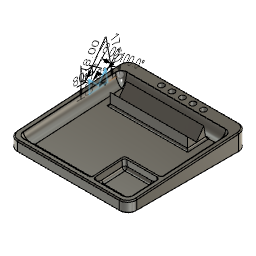
Rolling Tray with Mixer (Autodesk Fusion 360 design; units mm, degrees)
Autodesk Fusion 360 part; units mm, degrees
sketch "Esquisse2" plane through (0, 0, 0) normal (1, 0, 0) x (0, 1, 0)
  line L0 (0, 0) -> (170, 0)
  line L1 (170, 0) -> (170, 25)
  line L2 (0, 0) -> (0, 15)
  line L3 (170, 25) -> (0, 15)
  dimension "d3" = 170
  dimension "d4" = 15
  constraint coincident L0.start L2.start
  constraint horizontal L0
  constraint perpendicular L0 L1
  constraint vertical L2
  measures "d3" distance of L0.start L0.end
  measures "d4" distance of L0.start L2.end
extrude "Extrusion1" add sketch "Esquisse2" along normal blind 170
fillet "Congé1" radius 12.5 4 edges at (0, 170, 12.5) (0, 0, 7.5) (170, 0, 7.5) (170, 170, 12.5)
chamfer "Chanfrein1" distance 1.5 angle 45 16 edges at (85, 170, 25) (166.3388, 166.3388, 24.7846) (170, 85, 20) (166.3388, 3.6612, 15.2154) (85, 0, 15) (3.6612, 3.6612, 15.2154) (0, 85, 20) (3.6612, 166.3388, 24.7846) (0, 85, 0) (3.6612, 166.3388, 0) (85, 170, 0) (166.3388, 166.3388, 0) (170, 85, 0) (166.3388, 3.6612, 0) (85, 0, 0) (3.6612, 3.6612, 0)
sketch "Esquisse3" plane through (0, -0.8793, 14.9483) normal (0, -0.058722, 0.998274) x (1, 0, 0)
  line L0 (1.5, 158.5649) -> (1.5, 13.4024)
  spline S0 degree 3 poles (1.5003, 13.3248) (1.5002, 13.3377) (1.5001, 13.3506) (1.5, 13.3765) (1.5, 13.3895) (1.5, 13.4024) knots 1.56375 1.56375 1.56375 1.56375 1.567273 1.567273 1.570796 1.570796 1.570796 1.570796
  spline S1 degree 3 poles (12.5, 2.3808) (10.7152, 2.3808) (8.932, 2.8244) (6.3871, 4.174) (5.4968, 4.8327) (4.7227, 5.6081) (3.9487, 6.3835) (3.291, 7.2754) (1.9553, 9.8029) (1.5127, 11.5616) (1.5003, 13.3248) knots 0 0 0 0 0.486881 0.486881 0.785398 0.785398 0.785398 1.083915 1.083915 1.56375 1.56375 1.56375 1.56375
  line L1 (12.5, 2.3808) -> (157.5, 2.3808)
  spline S2 degree 3 poles (168.4997, 13.3248) (168.4873, 11.5616) (168.0447, 9.8029) (166.709, 7.2754) (166.0513, 6.3835) (165.2773, 5.6081) (164.5032, 4.8327) (163.6129, 4.174) (161.068, 2.8244) (159.2848, 2.3808) (157.5, 2.3808) knots -1.56375 -1.56375 -1.56375 -1.56375 -1.083915 -1.083915 -0.785398 -0.785398 -0.785398 -0.486881 -0.486881 0 0 0 0
  spline S3 degree 3 poles (168.5, 13.4024) (168.5, 13.3895) (168.5, 13.3765) (168.4999, 13.3506) (168.4998, 13.3377) (168.4997, 13.3248) knots -1.570796 -1.570796 -1.570796 -1.570796 -1.567273 -1.567273 -1.56375 -1.56375 -1.56375 -1.56375
  line L2 (168.5, 13.4024) -> (168.5, 158.5649)
  line L3 (168.5, 158.6531) -> (168.5, 158.5649)
  spline S4 degree 3 poles (157.5, 169.6747) (159.2794, 169.6747) (161.0571, 169.2338) (163.6041, 167.888) (164.4993, 167.2267) (165.2773, 166.4475) (166.0552, 165.6682) (166.7155, 164.7712) (168.0595, 162.2188) (168.5, 160.4367) (168.5, 158.6531) knots 0 0 0 0 0.485398 0.485398 0.785398 0.785398 0.785398 1.085399 1.085399 1.570796 1.570796 1.570796 1.570796
  line L4 (157.5, 169.6747) -> (12.5, 169.6747)
  spline S5 degree 3 poles (1.5, 158.6531) (1.5, 160.4367) (1.9405, 162.2188) (3.2845, 164.7712) (3.9448, 165.6682) (4.7227, 166.4475) (5.5007, 167.2267) (6.3959, 167.888) (8.9429, 169.2338) (10.7206, 169.6747) (12.5, 169.6747) knots -1.570796 -1.570796 -1.570796 -1.570796 -1.085399 -1.085399 -0.785398 -0.785398 -0.785398 -0.485398 -0.485398 0 0 0 0
  line L5 (1.5, 158.5649) -> (1.5, 158.6531)
  line L6 (163.5, 7.3808) -> (6.5, 7.3808)
  line L7 (6.5, 7.3808) -> (6.5, 154.6747)
  line L8 (6.5, 154.6747) -> (163.5, 154.6747)
  line L9 (163.5, 154.6747) -> (163.5, 7.3808)
  line L10 (163.5, 7.3808) -> (6.5, 154.6747) construction
  line L11 (6.5, 7.3808) -> (163.5, 154.6747) construction
  point P0 (85, 81.0278)
  dimension "d10" = 5
  dimension "d11" = 5
  dimension "d12" = 5
  dimension "d13" = 15
  constraint horizontal L6
  constraint perpendicular L6 L7
  constraint parallel L6 L8
  constraint parallel L7 L9
  constraint coincident L10 P0
  constraint coincident L11 P0
  measures "d10" distance of L1 L6
  measures "d11" distance of L2 L9
  measures "d12" distance of L0 L7
  measures "d13" distance of L4 L8
extrude "Extrusion2" cut sketch "Esquisse3" against normal blind 12.5 contours L6 L7 L8 L9
fillet "Congé2" radius 8 4 edges at (163.5, 153.8955, 17.7919) (163.5, 6.8558, 9.1425) (6.5, 6.8558, 9.1425) (6.5, 153.8955, 17.7919)
fillet "Congé4" radius 12 8 edges at (8.8431, 9.5619, 3.0409) (6.5, 80.7427, 7.228) (8.8431, 151.9234, 11.4151) (85, 154.2625, 11.5527) (161.1569, 151.9234, 11.4151) (163.5, 80.7427, 7.228) (161.1569, 9.5619, 3.0409) (85, 7.2228, 2.9033)
sketch "Esquisse5" plane through (0, 0, 0) normal (0, 0, -1) x (1, 0, 0)
  line L0 (1.5, -12.5) -> (1.5, -157.5)
  arc A0 (1.5, -157.5) -> (12.5, -168.5) centre (12.5, -157.5) ccw
  line L1 (12.5, -168.5) -> (157.5, -168.5)
  arc A1 (157.5, -168.5) -> (168.5, -157.5) centre (157.5, -157.5) ccw
  line L2 (168.5, -157.5) -> (168.5, -12.5)
  arc A2 (168.5, -12.5) -> (157.5, -1.5) centre (157.5, -12.5) ccw
  line L3 (157.5, -1.5) -> (12.5, -1.5)
  arc A3 (12.5, -1.5) -> (1.5, -12.5) centre (12.5, -12.5) ccw
  circle A4 centre (86.5, -161) radius 4
  circle A5 centre (101.5, -161) radius 4
  circle A6 centre (71.5, -161) radius 4
  circle A7 centre (116.5, -161) radius 4
  circle A8 centre (56.5, -161) radius 4
  dimension "d60" = 8
  dimension "d67" = 8
  dimension "d68" = 8
  dimension "d69" = 8
  dimension "d70" = 8
  measures "d60" diameter of A4
  measures "d67" diameter of A5
  measures "d68" diameter of A6
  measures "d69" diameter of A7
  measures "d70" diameter of A8
extrude "Extrusion3" cut sketch "Esquisse5" against normal blind 15 from surface at -10 contours A4 | A5 | A6 | A7 | A8
sketch "Esquisse6" plane through (0, 0, 0) normal (1, 0, 0) x (0, 1, 0)
  line L0 (140.9646, 10.5002) -> (137.9258, 27.7343)
  line L1 (140.9646, 10.5002) -> (159.1172, 10.5002) construction
  line L2 (137.9258, 27.7343) -> (127.6014, 12.9896)
  line L3 (127.6014, 12.9896) -> (114.8735, 25.7175)
  line L4 (114.8735, 25.7175) -> (114.8735, 8.2175)
  line L5 (140.9646, 10.5002) -> (114.8735, 8.2175)
  dimension "d47" = 100
  dimension "d48" = 80
  dimension "d49" = 45
  dimension "d50" = 17.5
  dimension "d51" = 17.5
  dimension "d52" = 18
  dimension "d53" = 18
  constraint horizontal L1
  constraint vertical L4
  measures "d47" angle of L0 L1
  measures "d48" angle of L2 L3
  measures "d49" angle of L0 L2
  measures "d50" distance of L0.start L0.end
  measures "d51" distance of L3.end L4.end
  measures "d52" distance of L0.end L2.end
  measures "d53" distance of L2.end L3.end
extrude "Extrusion4" add sketch "Esquisse6" along normal blind 110 from surface at 30
fillet "Congé5" radius 2.5 4 edges at (85, 114.8735, 9.2357) (140, 127.8955, 10.0017) (85, 140.9175, 10.7677) (30, 127.8955, 10.0017)
sketch "Esquisse8" plane through (0, -0.8793, 14.9483) normal (0, -0.058722, 0.998274) x (1, 0, 0)
  ellipse E0 centre (56.5, 162.1591) end of major axis (56.5, 166.1661) minor radius 4
  ellipse E1 centre (71.5, 162.1591) end of major axis (71.5, 166.1661) minor radius 4
  ellipse E2 centre (101.5, 162.1591) end of major axis (101.5, 166.1661) minor radius 4
  ellipse E3 centre (86.5, 162.1591) end of major axis (86.5, 166.1661) minor radius 4
  ellipse E4 centre (116.5, 162.1591) end of major axis (116.5, 166.1661) minor radius 4
  line L0 (6.5, 15.3808) -> (6.5, 146.6747)
  arc A0 (14.5, 154.6747) -> (6.5, 146.6747) centre (14.5, 146.6747) ccw
  line L1 (14.5, 154.6747) -> (155.5, 154.6747)
  arc A1 (163.5, 146.6747) -> (155.5, 154.6747) centre (155.5, 146.6747) ccw
  line L2 (163.5, 146.6747) -> (163.5, 15.3808)
  arc A2 (155.5, 7.3808) -> (163.5, 15.3808) centre (155.5, 15.3808) ccw
  line L3 (155.5, 7.3808) -> (14.5, 7.3808)
  arc A3 (6.5, 15.3808) -> (14.5, 7.3808) centre (14.5, 15.3808) ccw
  line L4 (1.5, 158.5649) -> (1.5, 13.4024)
  spline S0 degree 3 poles (1.5003, 13.3248) (1.5002, 13.3377) (1.5001, 13.3506) (1.5, 13.3765) (1.5, 13.3895) (1.5, 13.4024) knots 1.56375 1.56375 1.56375 1.56375 1.567273 1.567273 1.570796 1.570796 1.570796 1.570796
  spline S1 degree 3 poles (12.5, 2.3808) (10.7152, 2.3808) (8.932, 2.8244) (6.3871, 4.174) (5.4968, 4.8327) (4.7227, 5.6081) (3.9487, 6.3835) (3.291, 7.2754) (1.9553, 9.8029) (1.5127, 11.5616) (1.5003, 13.3248) knots 0 0 0 0 0.486881 0.486881 0.785398 0.785398 0.785398 1.083915 1.083915 1.56375 1.56375 1.56375 1.56375
  line L5 (12.5, 2.3808) -> (157.5, 2.3808)
  spline S2 degree 3 poles (168.4997, 13.3248) (168.4873, 11.5616) (168.0447, 9.8029) (166.709, 7.2754) (166.0513, 6.3835) (165.2773, 5.6081) (164.5032, 4.8327) (163.6129, 4.174) (161.068, 2.8244) (159.2848, 2.3808) (157.5, 2.3808) knots -1.56375 -1.56375 -1.56375 -1.56375 -1.083915 -1.083915 -0.785398 -0.785398 -0.785398 -0.486881 -0.486881 0 0 0 0
  spline S3 degree 3 poles (168.5, 13.4024) (168.5, 13.3895) (168.5, 13.3765) (168.4999, 13.3506) (168.4998, 13.3377) (168.4997, 13.3248) knots -1.570796 -1.570796 -1.570796 -1.570796 -1.567273 -1.567273 -1.56375 -1.56375 -1.56375 -1.56375
  line L6 (168.5, 13.4024) -> (168.5, 158.5649)
  line L7 (168.5, 158.6531) -> (168.5, 158.5649)
  spline S4 degree 3 poles (157.5, 169.6747) (159.2794, 169.6747) (161.0571, 169.2338) (163.6041, 167.888) (164.4993, 167.2267) (165.2773, 166.4475) (166.0552, 165.6682) (166.7155, 164.7712) (168.0595, 162.2188) (168.5, 160.4367) (168.5, 158.6531) knots 0 0 0 0 0.485398 0.485398 0.785398 0.785398 0.785398 1.085399 1.085399 1.570796 1.570796 1.570796 1.570796
  line L8 (157.5, 169.6747) -> (12.5, 169.6747)
  spline S5 degree 3 poles (1.5, 158.6531) (1.5, 160.4367) (1.9405, 162.2188) (3.2845, 164.7712) (3.9448, 165.6682) (4.7227, 166.4475) (5.5007, 167.2267) (6.3959, 167.888) (8.9429, 169.2338) (10.7206, 169.6747) (12.5, 169.6747) knots -1.570796 -1.570796 -1.570796 -1.570796 -1.085399 -1.085399 -0.785398 -0.785398 -0.785398 -0.485398 -0.485398 0 0 0 0
  line L9 (1.5, 158.5649) -> (1.5, 158.6531)
  line L10 (163.5, 52.3808) -> (113.5, 52.3808)
  line L11 (113.5, 52.3808) -> (113.5, 54.8808)
  line L12 (113.5, 54.8808) -> (163.5, 54.8808)
  line L13 (163.5, 54.8808) -> (163.5, 52.3808)
  line L14 (113.5, 54.8808) -> (111, 54.8808)
  line L15 (111, 54.8808) -> (111, 7.3808)
  line L16 (111, 7.3808) -> (113.5, 7.3808)
  line L17 (113.5, 7.3808) -> (113.5, 54.8808)
  dimension "d71" = 50
  dimension "d72" = 2.5
  dimension "d73" = 45
  dimension "d74" = 2.5
  constraint horizontal L10
  constraint vertical L11
  constraint horizontal L12
  constraint vertical L13
  constraint coincident L2 L10.start
  constraint horizontal L14
  constraint vertical L15
  constraint horizontal L16
  constraint vertical L17
  constraint coincident L3 L15.end
  measures "d71" distance of L11.end L12.end
  measures "d72" distance of L10.end L11.end
  measures "d73" distance of L3 L10
  measures "d74" distance of L11.end L14.end
extrude "Extrusion5" add sketch "Esquisse8" against normal blind 15 contours L3 L11 L14 L15 L16 L17 | L2 L10 L11 L12 L13 L17
fillet "Congé8" radius 3.5 14 edges at (113.5, 51.7781, 11.785) (163.5, 51.4258, 17.7746) (159.9853, 51.9388, 9.0544) (132.5, 52.1452, 5.5458) (131.25, 54.6408, 5.6926) (159.9853, 54.4345, 9.2012) (163.5, 53.9215, 17.9214) (111, 54.2738, 11.9318) (111, 6.5035, 15.1321) (111, 10.5251, 6.6183) (111, 36.9215, 4.6502) (113.5, 35.6736, 4.5768) (113.5, 10.5251, 6.6183) (113.5, 6.5035, 15.1321)
